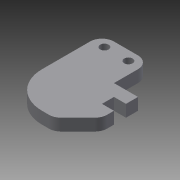
# Autodesk Inventor part: holdBar
Saved by Autodesk Inventor 2015 (Build 190159000, 159)
## iProperties
Created: 2016-10-14
Part Number: holdBar
Material: Generic
Document SubType Name: Modeling
Designer: Bardo91
Density: 1 g/cm^3
Appearance: Default
Author: Bardo91
Autodesk Inventor part; units mm, degrees
ref_plane "YZ Plane" through (0, 0, 0) normal (1, 0, 0) x (0, 1, 0)
ref_plane "XZ Plane" through (0, 0, 0) normal (0, 1, 0) x (-1, 0, 0)
ref_plane "XY Plane" through (0, 0, 0) normal (0, 0, 1) x (1, 0, 0)
sketch "Sketch1" plane through (0, 0, 0) normal (0, 0, 1) x (1, 0, 0)
  line L0 (0, 0) -> (-10, 0)
  line L1 (-10, 0) -> (-10, 5)
  line L2 (-5, 10) -> (5, 10)
  line L3 (10, 5) -> (10, -5)
  line L4 (10, -5) -> (20, -5)
  line L5 (20, -5) -> (20, -10)
  line L6 (20, -10) -> (10, -10)
  line L7 (10, -10) -> (10, -15)
  line L8 (10, -15) -> (20, -15)
  line L9 (20, -15) -> (20, -17.9289)
  line L10 (18.5355, -21.4645) -> (11.4645, -28.5355)
  line L11 (7.9289, -30) -> (5, -30)
  line L12 (-10, -15) -> (-10, 0)
  arc A0 (-5, 10) -> (-10, 5) centre (-5, 5) ccw
  arc A1 (10, 5) -> (5, 10) centre (5, 5) ccw
  arc A2 (-10, -15) -> (5, -30) centre (5, -15) ccw
  arc A3 (7.9289, -30) -> (11.4645, -28.5355) centre (7.9289, -25) ccw
  arc A4 (18.5355, -21.4645) -> (20, -17.9289) centre (15, -17.9289) ccw
  line L13 (10, -10) -> (15, -10)
  line L14 (15, -10) -> (15, -15)
  point P0 (-10, 10)
  point P1 (10, 10)
  point P2 (20, -20)
  point P3 (10, -30)
  dimension "d0" = 10
  dimension "d1" = 10
  dimension "d2" = 20
  dimension "d3" = 15
  dimension "d4" = 10
  dimension "d5" = 5
  dimension "d6" = 5
  dimension "d7" = 5
  dimension "d8" = 135
  dimension "d9" = 5
  dimension "d10" = 15
  dimension "d11" = 5
  dimension "d21" = 5
  constraints: 30 end point, 13 point on line, 10 point on circle, 10 tangent, 7 perpendicular, 5 centre point, 2 equal radius, 2 horizontal, 2 midpoint, 1 parallel
  measures "d0" distance of L0.start L0.end
  measures "d1" distance of L0.end point (-10, 10)
  measures "d2" distance of point (-10, 10) point (10, 10)
  measures "d3" distance of point (10, 10) L3.end
  measures "d4" distance of L3.end L4.end
  measures "d5" distance of L4.end L5.end
  measures "d6" distance of L6.end L7.end
  measures "d7" distance of L8.end point (20, -20)
  measures "d8" angle of L9 L10
  measures "d9" radius of A0
  measures "d10" radius of A2
  measures "d11" radius of A3
  measures "d21" distance of L6.end L13.end
extrude "Extrusion1" add sketch "Sketch1" along normal blind 5
sketch "Sketch2" plane through (0, 0, 5) normal (0, 0, 1) x (1, 0, 0)
  line L0 (0, 0) -> (0, 6)
  line L1 (0, 6) -> (5, 6)
  line L2 (5, 6) -> (-5, 6)
  circle A0 centre (-5, 6) radius 1.75
  circle A1 centre (5, 6) radius 1.75
  dimension "d14" = 6
  dimension "d15" = 5
  dimension "d16" = 10
  dimension "d17" = 3.5
  dimension "d18" = 3.5
  constraints: 6 end point, 2 centre point, 2 coincident, 1 perpendicular, 1 point on line, 1 vertical
  measures "d14" distance of L0.start L0.end
  measures "d15" distance of L0.end L1.end
  measures "d16" distance of L1.end L2.end
  measures "d17" diameter of A0
  measures "d18" diameter of A1
extrude "Extrusion2" cut sketch "Sketch2" against normal blind 5
body "Solid1"
